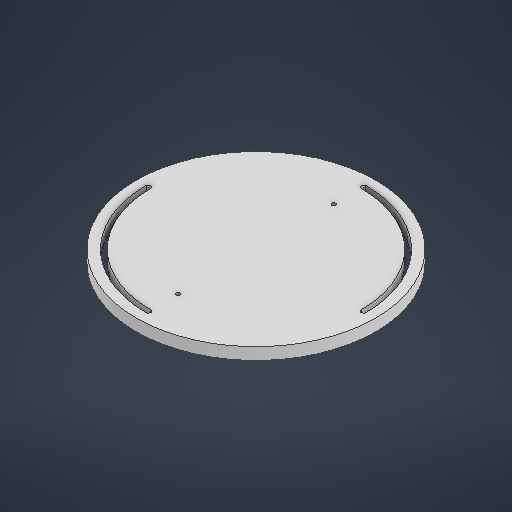
# Autodesk Inventor part: Aufhängung_Drehscheibe
Saved by Autodesk Inventor 2027 (Build 310192060, 192F)
## iProperties
Created: 2026-07-23
Part Number: Aufhängung_Drehscheibe
Material: Generic
Document SubType Name: Modeling
Designer: kw
Density: 1 g/cm^3
Appearance: Default
Author: kw
Autodesk Inventor part; units mm, degrees
ref_plane "YZ Plane" through (0, 0, 0) normal (1, 0, 0) x (0, 1, 0)
ref_plane "XZ Plane" through (0, 0, 0) normal (0, 1, 0) x (-1, 0, 0)
ref_plane "XY Plane" through (0, 0, 0) normal (0, 0, 1) x (1, 0, 0)
sketch "Sketch1" plane through (0, 0, 0) normal (0, 1, 0) x (-1, 0, 0)
  circle A0 centre (0, 0) radius 100
  circle A1 centre (0, 0) radius 80
  circle A2 centre (0, 0) radius 90
  circle A3 centre (0, 0) radius 88
  circle A4 centre (0, 0) radius 92
  arc A5 (88, 0) -> (92, 0) centre (90, 0) ccw
  arc A6 (0, 92) -> (0, 88) centre (0, 90) ccw
  arc A7 (-88, 0) -> (-92, 0) centre (-90, 0) ccw
  arc A8 (0, -92) -> (0, -88) centre (0, -90) ccw
  dimension "d0" = 200
  dimension "d3" = 20
  dimension "d4" = 10
  dimension "d5" = 2
  dimension "d6" = 2
  constraints: 16 point on circle, 9 centre point, 8 tangent, 1 coincident
  measures "d0" diameter of A0
  measures "d3" radial gap between concentric circles of A0 A1
  measures "d4" radial gap between concentric circles of A0 A2
  measures "d5" radial gap between concentric circles of A2 A3
  measures "d6" radial gap between concentric circles of A2 A4
extrude "Extrusion1" add sketch "Sketch1" along normal blind 10 contours A0 | A1 | A6 A3 A7 A2 | A2 A7 A4 A6 | A5 A4 A8 A2 | A2 A8 A3 A5 | A3
sketch "Sketch2" plane through (0, 10, 0) normal (0, 1, 0) x (1, 0, 0)
  line L0 (0, 0) -> (0, -65)
  line L1 (0, -65) -> (0, 65)
  dimension "d7" = 65
  dimension "d8" = 130
  constraints: 4 end point, 1 point on line, 1 vertical
  measures "d7" distance of L0.start L0.end
  measures "d8" distance of L0.end L1.end
hole "Hole1" at (0, 10, 65) at (0, 10, -65) direction (0, -1, 0) diameter 3.242 end through all thread size "M4x0.7" class "6H" standard "ISO Metric profile"
body "Solid1"
